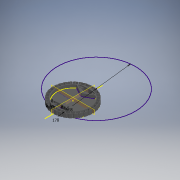
# Autodesk Inventor part: tsop_lid_edge
Saved by Autodesk Inventor 2020 (Build 240168000, 168)
## iProperties
Created: 2024-11-04
Part Number: tsop_lid_edge
Material: Полиэтилен, низкая плотность
Document SubType Name: Modeling
Designer: Ivan
Density: 0.894 g/cm^3
Appearance: Типовые
Mass: 25.9843 g
Surface Area: 265.893 cm^2
Volume: 29.0652 cm^3
Author: Ivan
Autodesk Inventor part; units mm, degrees
ref_plane "XZ Plane" through (0, 0, 0) normal (0, 1, 0) x (-1, 0, 0)
sketch "Эскиз1" plane through (0, 0, 0) normal (0, 1, 0) x (-1, 0, 0)
  line L0 (44.0469, 3.6) -> (38.8469, 3.6)
  line L1 (38.8469, 3.6) -> (38.8469, -3.6)
  line L2 (38.8469, -3.6) -> (44.0469, -3.6)
  line L3 (44.0469, -3.6) -> (44.0469, 3.6)
  line L4 (0, 0) -> (38.8469, 0) construction
  circle A0 centre (0, 0) radius 41.603 construction
  line L5 (41.4469, 3.6) -> (41.4469, -3.6) construction
  line L6 (37.3982, 11.1095) -> (38.8028, 4.0478)
  line L7 (42.4983, 12.124) -> (37.3982, 11.1095)
  line L8 (43.9029, 5.0623) -> (42.4983, 12.124)
  line L9 (38.8028, 4.0478) -> (43.9029, 5.0623)
  line L10 (34.5122, 18.192) -> (37.2675, 11.5401)
  line L11 (39.3164, 20.182) -> (34.5122, 18.192)
  line L12 (42.0717, 13.5301) -> (39.3164, 20.182)
  line L13 (37.2675, 11.5401) -> (42.0717, 13.5301)
  line L14 (30.3, 24.5755) -> (34.3001, 18.5889)
  line L15 (34.6236, 27.4645) -> (30.3, 24.5755)
  line L16 (38.6237, 21.4779) -> (34.6236, 27.4645)
  line L17 (34.3001, 18.5889) -> (38.6237, 21.4779)
  line L18 (24.9233, 30.0145) -> (30.0145, 24.9233)
  line L19 (28.6003, 33.6915) -> (24.9233, 30.0145)
  line L20 (33.6915, 28.6003) -> (28.6003, 33.6915)
  line L21 (30.0145, 24.9233) -> (33.6915, 28.6003)
  line L22 (18.5889, 34.3001) -> (24.5755, 30.3)
  line L23 (21.4779, 38.6237) -> (18.5889, 34.3001)
  line L24 (27.4645, 34.6236) -> (21.4779, 38.6237)
  line L25 (24.5755, 30.3) -> (27.4645, 34.6236)
  line L26 (11.5401, 37.2675) -> (18.192, 34.5122)
  line L27 (13.5301, 42.0717) -> (11.5401, 37.2675)
  line L28 (20.182, 39.3164) -> (13.5301, 42.0717)
  line L29 (18.192, 34.5122) -> (20.182, 39.3164)
  line L30 (4.0478, 38.8028) -> (11.1095, 37.3982)
  line L31 (5.0623, 43.9029) -> (4.0478, 38.8028)
  line L32 (12.124, 42.4983) -> (5.0623, 43.9029)
  line L33 (11.1095, 37.3982) -> (12.124, 42.4983)
  line L34 (-3.6, 38.8469) -> (3.6, 38.8469)
  line L35 (-3.6, 44.0469) -> (-3.6, 38.8469)
  line L36 (3.6, 44.0469) -> (-3.6, 44.0469)
  line L37 (3.6, 38.8469) -> (3.6, 44.0469)
  line L38 (-11.1095, 37.3982) -> (-4.0478, 38.8028)
  line L39 (-12.124, 42.4983) -> (-11.1095, 37.3982)
  line L40 (-5.0623, 43.9029) -> (-12.124, 42.4983)
  line L41 (-4.0478, 38.8028) -> (-5.0623, 43.9029)
  line L42 (-18.192, 34.5122) -> (-11.5401, 37.2675)
  line L43 (-20.182, 39.3164) -> (-18.192, 34.5122)
  line L44 (-13.5301, 42.0717) -> (-20.182, 39.3164)
  line L45 (-11.5401, 37.2675) -> (-13.5301, 42.0717)
  line L46 (-24.5755, 30.3) -> (-18.5889, 34.3001)
  line L47 (-27.4645, 34.6236) -> (-24.5755, 30.3)
  line L48 (-21.4779, 38.6237) -> (-27.4645, 34.6236)
  line L49 (-18.5889, 34.3001) -> (-21.4779, 38.6237)
  line L50 (-30.0145, 24.9233) -> (-24.9233, 30.0145)
  line L51 (-33.6915, 28.6003) -> (-30.0145, 24.9233)
  line L52 (-28.6003, 33.6915) -> (-33.6915, 28.6003)
  line L53 (-24.9233, 30.0145) -> (-28.6003, 33.6915)
  line L54 (-34.3001, 18.5889) -> (-30.3, 24.5755)
  line L55 (-38.6237, 21.4779) -> (-34.3001, 18.5889)
  line L56 (-34.6236, 27.4645) -> (-38.6237, 21.4779)
  line L57 (-30.3, 24.5755) -> (-34.6236, 27.4645)
  line L58 (-37.2675, 11.5401) -> (-34.5122, 18.192)
  line L59 (-42.0717, 13.5301) -> (-37.2675, 11.5401)
  line L60 (-39.3164, 20.182) -> (-42.0717, 13.5301)
  line L61 (-34.5122, 18.192) -> (-39.3164, 20.182)
  line L62 (-38.8028, 4.0478) -> (-37.3982, 11.1095)
  line L63 (-43.9029, 5.0623) -> (-38.8028, 4.0478)
  line L64 (-42.4983, 12.124) -> (-43.9029, 5.0623)
  line L65 (-37.3982, 11.1095) -> (-42.4983, 12.124)
  line L66 (-38.8469, -3.6) -> (-38.8469, 3.6)
  line L67 (-44.0469, -3.6) -> (-38.8469, -3.6)
  line L68 (-44.0469, 3.6) -> (-44.0469, -3.6)
  line L69 (-38.8469, 3.6) -> (-44.0469, 3.6)
  line L70 (-37.3982, -11.1095) -> (-38.8028, -4.0478)
  line L71 (-42.4983, -12.124) -> (-37.3982, -11.1095)
  line L72 (-43.9029, -5.0623) -> (-42.4983, -12.124)
  line L73 (-38.8028, -4.0478) -> (-43.9029, -5.0623)
  line L74 (-34.5122, -18.192) -> (-37.2675, -11.5401)
  line L75 (-39.3164, -20.182) -> (-34.5122, -18.192)
  line L76 (-42.0717, -13.5301) -> (-39.3164, -20.182)
  line L77 (-37.2675, -11.5401) -> (-42.0717, -13.5301)
  line L78 (-30.3, -24.5755) -> (-34.3001, -18.5889)
  line L79 (-34.6236, -27.4645) -> (-30.3, -24.5755)
  line L80 (-38.6237, -21.4779) -> (-34.6236, -27.4645)
  line L81 (-34.3001, -18.5889) -> (-38.6237, -21.4779)
  line L82 (-24.9233, -30.0145) -> (-30.0145, -24.9233)
  line L83 (-28.6003, -33.6915) -> (-24.9233, -30.0145)
  line L84 (-33.6915, -28.6003) -> (-28.6003, -33.6915)
  line L85 (-30.0145, -24.9233) -> (-33.6915, -28.6003)
  line L86 (-18.5889, -34.3001) -> (-24.5755, -30.3)
  line L87 (-21.4779, -38.6237) -> (-18.5889, -34.3001)
  line L88 (-27.4645, -34.6236) -> (-21.4779, -38.6237)
  line L89 (-24.5755, -30.3) -> (-27.4645, -34.6236)
  line L90 (-11.5401, -37.2675) -> (-18.192, -34.5122)
  line L91 (-13.5301, -42.0717) -> (-11.5401, -37.2675)
  line L92 (-20.182, -39.3164) -> (-13.5301, -42.0717)
  line L93 (-18.192, -34.5122) -> (-20.182, -39.3164)
  line L94 (-4.0478, -38.8028) -> (-11.1095, -37.3982)
  line L95 (-5.0623, -43.9029) -> (-4.0478, -38.8028)
  line L96 (-12.124, -42.4983) -> (-5.0623, -43.9029)
  line L97 (-11.1095, -37.3982) -> (-12.124, -42.4983)
  line L98 (3.6, -38.8469) -> (-3.6, -38.8469)
  line L99 (3.6, -44.0469) -> (3.6, -38.8469)
  line L100 (-3.6, -44.0469) -> (3.6, -44.0469)
  line L101 (-3.6, -38.8469) -> (-3.6, -44.0469)
  line L102 (11.1095, -37.3982) -> (4.0478, -38.8028)
  line L103 (12.124, -42.4983) -> (11.1095, -37.3982)
  line L104 (5.0623, -43.9029) -> (12.124, -42.4983)
  line L105 (4.0478, -38.8028) -> (5.0623, -43.9029)
  line L106 (18.192, -34.5122) -> (11.5401, -37.2675)
  line L107 (20.182, -39.3164) -> (18.192, -34.5122)
  line L108 (13.5301, -42.0717) -> (20.182, -39.3164)
  line L109 (11.5401, -37.2675) -> (13.5301, -42.0717)
  line L110 (24.5755, -30.3) -> (18.5889, -34.3001)
  line L111 (27.4645, -34.6236) -> (24.5755, -30.3)
  line L112 (21.4779, -38.6237) -> (27.4645, -34.6236)
  line L113 (18.5889, -34.3001) -> (21.4779, -38.6237)
  line L114 (30.0145, -24.9233) -> (24.9233, -30.0145)
  line L115 (33.6915, -28.6003) -> (30.0145, -24.9233)
  line L116 (28.6003, -33.6915) -> (33.6915, -28.6003)
  line L117 (24.9233, -30.0145) -> (28.6003, -33.6915)
  line L118 (34.3001, -18.5889) -> (30.3, -24.5755)
  line L119 (38.6237, -21.4779) -> (34.3001, -18.5889)
  line L120 (34.6236, -27.4645) -> (38.6237, -21.4779)
  line L121 (30.3, -24.5755) -> (34.6236, -27.4645)
  line L122 (37.2675, -11.5401) -> (34.5122, -18.192)
  line L123 (42.0717, -13.5301) -> (37.2675, -11.5401)
  line L124 (39.3164, -20.182) -> (42.0717, -13.5301)
  line L125 (34.5122, -18.192) -> (39.3164, -20.182)
  line L126 (38.8028, -4.0478) -> (37.3982, -11.1095)
  line L127 (43.9029, -5.0623) -> (38.8028, -4.0478)
  line L128 (42.4983, -12.124) -> (43.9029, -5.0623)
  line L129 (37.3982, -11.1095) -> (42.4983, -12.124)
  line L130 (38.8028, 4.0478) -> (38.8469, 3.6) construction
  line L131 (38.8469, 3.6) -> (43.9777, 4.1053) construction
  line L132 (43.9029, 5.0623) -> (37.3982, 11.1095) construction
  line L133 (42.4983, 12.124) -> (38.8028, 4.0478) construction
  circle A1 centre (0, 0) radius 41.4469 construction
  line L134 (39.3164, 20.182) -> (37.2675, 11.5401) construction
  line L135 (34.5122, 18.192) -> (42.0717, 13.5301) construction
  line L136 (38.292, 15.8611) -> (0, 0) construction
  line L137 (0, 0) -> (40.6505, 8.0859) construction
  point P0 (41.603, 0)
  point P1 (38.1005, 7.5787)
  point P2 (39.9482, 11.6167)
  point P3 (41.3529, 4.5551)
  point P4 (35.8899, 14.8661)
  point P5 (36.9143, 19.187)
  point P6 (39.6696, 12.5351)
  point P7 (32.3, 21.5822)
  point P8 (32.4618, 26.02)
  point P9 (36.4619, 20.0334)
  point P10 (27.4689, 27.4689)
  point P11 (26.7618, 31.853)
  point P12 (31.853, 26.7618)
  point P13 (21.5822, 32.3)
  point P14 (20.0334, 36.4619)
  point P15 (26.02, 32.4618)
  point P16 (14.8661, 35.8899)
  point P17 (12.5351, 39.6696)
  point P18 (19.187, 36.9143)
  point P19 (7.5787, 38.1005)
  point P20 (4.5551, 41.3529)
  point P21 (11.6167, 39.9482)
  point P22 (0, 38.8469)
  point P23 (-3.6, 41.4469)
  point P24 (3.6, 41.4469)
  point P25 (-7.5787, 38.1005)
  point P26 (-11.6167, 39.9482)
  point P27 (-4.5551, 41.3529)
  point P28 (-14.8661, 35.8899)
  point P29 (-19.187, 36.9143)
  point P30 (-12.5351, 39.6696)
  point P31 (-21.5822, 32.3)
  point P32 (-26.02, 32.4618)
  point P33 (-20.0334, 36.4619)
  point P34 (-27.4689, 27.4689)
  point P35 (-31.853, 26.7618)
  point P36 (-26.7618, 31.853)
  point P37 (-32.3, 21.5822)
  point P38 (-36.4619, 20.0334)
  point P39 (-32.4618, 26.02)
  point P40 (-35.8899, 14.8661)
  point P41 (-39.6696, 12.5351)
  point P42 (-36.9143, 19.187)
  point P43 (-38.1005, 7.5787)
  point P44 (-41.3529, 4.5551)
  point P45 (-39.9482, 11.6167)
  point P46 (-38.8469, 0)
  point P47 (-41.4469, -3.6)
  point P48 (-41.4469, 3.6)
  point P49 (-38.1005, -7.5787)
  point P50 (-39.9482, -11.6167)
  point P51 (-41.3529, -4.5551)
  point P52 (-35.8899, -14.8661)
  point P53 (-36.9143, -19.187)
  point P54 (-39.6696, -12.5351)
  point P55 (-32.3, -21.5822)
  point P56 (-32.4618, -26.02)
  point P57 (-36.4619, -20.0334)
  point P58 (-27.4689, -27.4689)
  point P59 (-26.7618, -31.853)
  point P60 (-31.853, -26.7618)
  point P61 (-21.5822, -32.3)
  point P62 (-20.0334, -36.4619)
  point P63 (-26.02, -32.4618)
  point P64 (-14.8661, -35.8899)
  point P65 (-12.5351, -39.6696)
  point P66 (-19.187, -36.9143)
  point P67 (-7.5787, -38.1005)
  point P68 (-4.5551, -41.3529)
  point P69 (-11.6167, -39.9482)
  point P70 (0, -38.8469)
  point P71 (3.6, -41.4469)
  point P72 (-3.6, -41.4469)
  point P73 (7.5787, -38.1005)
  point P74 (11.6167, -39.9482)
  point P75 (4.5551, -41.3529)
  point P76 (14.8661, -35.8899)
  point P77 (19.187, -36.9143)
  point P78 (12.5351, -39.6696)
  point P79 (21.5822, -32.3)
  point P80 (26.02, -32.4618)
  point P81 (20.0334, -36.4619)
  point P82 (27.4689, -27.4689)
  point P83 (31.853, -26.7618)
  point P84 (26.7618, -31.853)
  point P85 (32.3, -21.5822)
  point P86 (36.4619, -20.0334)
  point P87 (32.4618, -26.02)
  point P88 (35.8899, -14.8661)
  point P89 (39.6696, -12.5351)
  point P90 (36.9143, -19.187)
  point P91 (38.1005, -7.5787)
  point P92 (41.3529, -4.5551)
  point P93 (39.9482, -11.6167)
  dimension "d79" = 82.8939
  dimension "d0" = 7.2
  dimension "d1" = 5.2
  dimension "d5" = 360
  dimension "d7" = 0.45
  dimension "d80" = 7.2
  dimension "d81" = 5.2
  dimension "d82" = 11.25
  dimension "d83" = 11.25
  constraints: 274 end point, 35 midpoint, 3 point on circle, 2 coincident, 2 horizontal, 2 perpendicular, 1 centre point, 1 parallel, 1 point on line, 1 vertical, 360 other
  measures "d0" distance of L1.start L1.end
  measures "d1" distance from line of L1 L2.end
  measures "d7" distance from line of L131 L6.end
  measures "d80" distance between parallel lines of L9 L7
  measures "d81" distance between parallel lines of L6 L8
  measures "d82" angle to the sketch x axis of L9
  measures "d83" angle of L137 L136
sketch "Эскиз3" plane through (0, 0, 0) normal (0, 1, 0) x (-1, 0, 0)
  line L0 (38.8028, 4.0478) -> (38.8469, 3.6) construction
  line L1 (38.8249, 3.8239) -> (46.4311, 4.5731) construction
  line L2 (44.0469, -3.6) -> (44.0469, 3.6) projected
  line L3 (44.0469, -0.05) -> (44.0469, 0.05)
  line L4 (44.0469, 2.45) -> (45.2469, 2.45) construction
  arc A0 (44.0469, 0.05) -> (45.2469, 2.45) centre (42.2469, 2.45) ccw
  line L5 (45.2469, 2.45) -> (45.2469, 0) construction
  line L6 (0, 0) -> (38.8469, 0) construction
  arc A1 (45.2469, -2.45) -> (44.0469, -0.05) centre (42.2469, -2.45) ccw
  arc A2 (43.1908, 8.6422) -> (43.8996, 11.2302) centre (40.9572, 10.6449) ccw
  arc A3 (44.8555, 6.4243) -> (43.2103, 8.5441) centre (41.9131, 5.839) ccw
  line L7 (43.2103, 8.5441) -> (43.1908, 8.6422)
  arc A4 (40.6749, 16.9022) -> (40.8651, 19.5788) centre (38.0935, 18.4307) ccw
  arc A5 (42.7403, 15.0517) -> (40.7132, 16.8098) centre (39.9686, 13.9037) ccw
  line L8 (40.7132, 16.8098) -> (40.6749, 16.9022)
  arc A6 (36.5959, 24.5127) -> (36.2603, 27.1749) centre (33.7659, 25.5082) ccw
  arc A7 (38.9826, 23.1007) -> (36.6515, 24.4296) centre (36.4882, 21.434) ccw
  line L9 (36.6515, 24.4296) -> (36.5959, 24.5127)
  arc A8 (31.1105, 31.1812) -> (30.262, 33.7268) centre (28.1407, 31.6055) ccw
  arc A9 (33.7268, 30.262) -> (31.1812, 31.1105) centre (31.6055, 28.1407) ccw
  line L10 (31.1812, 31.1105) -> (31.1105, 31.1812)
  arc A10 (24.4296, 36.6515) -> (23.1007, 38.9826) centre (21.434, 36.4882) ccw
  arc A11 (27.1749, 36.2603) -> (24.5127, 36.5959) centre (25.5082, 33.7659) ccw
  line L11 (24.5127, 36.5959) -> (24.4296, 36.6515)
  arc A12 (16.8098, 40.7132) -> (15.0517, 42.7403) centre (13.9037, 39.9686) ccw
  arc A13 (19.5788, 40.8651) -> (16.9022, 40.6749) centre (18.4307, 38.0935) ccw
  line L12 (16.9022, 40.6749) -> (16.8098, 40.7132)
  arc A14 (8.5441, 43.2103) -> (6.4243, 44.8555) centre (5.839, 41.9131) ccw
  arc A15 (11.2302, 43.8996) -> (8.6422, 43.1908) centre (10.6449, 40.9572) ccw
  line L13 (8.6422, 43.1908) -> (8.5441, 43.2103)
  arc A16 (-0.05, 44.0469) -> (-2.45, 45.2469) centre (-2.45, 42.2469) ccw
  arc A17 (2.45, 45.2469) -> (0.05, 44.0469) centre (2.45, 42.2469) ccw
  line L14 (0.05, 44.0469) -> (-0.05, 44.0469)
  arc A18 (-8.6422, 43.1908) -> (-11.2302, 43.8996) centre (-10.6449, 40.9572) ccw
  arc A19 (-6.4243, 44.8555) -> (-8.5441, 43.2103) centre (-5.839, 41.9131) ccw
  line L15 (-8.5441, 43.2103) -> (-8.6422, 43.1908)
  arc A20 (-16.9022, 40.6749) -> (-19.5788, 40.8651) centre (-18.4307, 38.0935) ccw
  arc A21 (-15.0517, 42.7403) -> (-16.8098, 40.7132) centre (-13.9037, 39.9686) ccw
  line L16 (-16.8098, 40.7132) -> (-16.9022, 40.6749)
  arc A22 (-24.5127, 36.5959) -> (-27.1749, 36.2603) centre (-25.5082, 33.7659) ccw
  arc A23 (-23.1007, 38.9826) -> (-24.4296, 36.6515) centre (-21.434, 36.4882) ccw
  line L17 (-24.4296, 36.6515) -> (-24.5127, 36.5959)
  arc A24 (-31.1812, 31.1105) -> (-33.7268, 30.262) centre (-31.6055, 28.1407) ccw
  arc A25 (-30.262, 33.7268) -> (-31.1105, 31.1812) centre (-28.1407, 31.6055) ccw
  line L18 (-31.1105, 31.1812) -> (-31.1812, 31.1105)
  arc A26 (-36.6515, 24.4296) -> (-38.9826, 23.1007) centre (-36.4882, 21.434) ccw
  arc A27 (-36.2603, 27.1749) -> (-36.5959, 24.5127) centre (-33.7659, 25.5082) ccw
  line L19 (-36.5959, 24.5127) -> (-36.6515, 24.4296)
  arc A28 (-40.7132, 16.8098) -> (-42.7403, 15.0517) centre (-39.9686, 13.9037) ccw
  arc A29 (-40.8651, 19.5788) -> (-40.6749, 16.9022) centre (-38.0935, 18.4307) ccw
  line L20 (-40.6749, 16.9022) -> (-40.7132, 16.8098)
  arc A30 (-43.2103, 8.5441) -> (-44.8555, 6.4243) centre (-41.9131, 5.839) ccw
  arc A31 (-43.8996, 11.2302) -> (-43.1908, 8.6422) centre (-40.9572, 10.6449) ccw
  line L21 (-43.1908, 8.6422) -> (-43.2103, 8.5441)
  arc A32 (-44.0469, -0.05) -> (-45.2469, -2.45) centre (-42.2469, -2.45) ccw
  arc A33 (-45.2469, 2.45) -> (-44.0469, 0.05) centre (-42.2469, 2.45) ccw
  line L22 (-44.0469, 0.05) -> (-44.0469, -0.05)
  arc A34 (-43.1908, -8.6422) -> (-43.8996, -11.2302) centre (-40.9572, -10.6449) ccw
  arc A35 (-44.8555, -6.4243) -> (-43.2103, -8.5441) centre (-41.9131, -5.839) ccw
  line L23 (-43.2103, -8.5441) -> (-43.1908, -8.6422)
  arc A36 (-40.6749, -16.9022) -> (-40.8651, -19.5788) centre (-38.0935, -18.4307) ccw
  arc A37 (-42.7403, -15.0517) -> (-40.7132, -16.8098) centre (-39.9686, -13.9037) ccw
  line L24 (-40.7132, -16.8098) -> (-40.6749, -16.9022)
  arc A38 (-36.5959, -24.5127) -> (-36.2603, -27.1749) centre (-33.7659, -25.5082) ccw
  arc A39 (-38.9826, -23.1007) -> (-36.6515, -24.4296) centre (-36.4882, -21.434) ccw
  line L25 (-36.6515, -24.4296) -> (-36.5959, -24.5127)
  arc A40 (-31.1105, -31.1812) -> (-30.262, -33.7268) centre (-28.1407, -31.6055) ccw
  arc A41 (-33.7268, -30.262) -> (-31.1812, -31.1105) centre (-31.6055, -28.1407) ccw
  line L26 (-31.1812, -31.1105) -> (-31.1105, -31.1812)
  arc A42 (-24.4296, -36.6515) -> (-23.1007, -38.9826) centre (-21.434, -36.4882) ccw
  arc A43 (-27.1749, -36.2603) -> (-24.5127, -36.5959) centre (-25.5082, -33.7659) ccw
  line L27 (-24.5127, -36.5959) -> (-24.4296, -36.6515)
  arc A44 (-16.8098, -40.7132) -> (-15.0517, -42.7403) centre (-13.9037, -39.9686) ccw
  arc A45 (-19.5788, -40.8651) -> (-16.9022, -40.6749) centre (-18.4307, -38.0935) ccw
  line L28 (-16.9022, -40.6749) -> (-16.8098, -40.7132)
  arc A46 (-8.5441, -43.2103) -> (-6.4243, -44.8555) centre (-5.839, -41.9131) ccw
  arc A47 (-11.2302, -43.8996) -> (-8.6422, -43.1908) centre (-10.6449, -40.9572) ccw
  line L29 (-8.6422, -43.1908) -> (-8.5441, -43.2103)
  arc A48 (0.05, -44.0469) -> (2.45, -45.2469) centre (2.45, -42.2469) ccw
  arc A49 (-2.45, -45.2469) -> (-0.05, -44.0469) centre (-2.45, -42.2469) ccw
  line L30 (-0.05, -44.0469) -> (0.05, -44.0469)
  arc A50 (8.6422, -43.1908) -> (11.2302, -43.8996) centre (10.6449, -40.9572) ccw
  arc A51 (6.4243, -44.8555) -> (8.5441, -43.2103) centre (5.839, -41.9131) ccw
  line L31 (8.5441, -43.2103) -> (8.6422, -43.1908)
  arc A52 (16.9022, -40.6749) -> (19.5788, -40.8651) centre (18.4307, -38.0935) ccw
  arc A53 (15.0517, -42.7403) -> (16.8098, -40.7132) centre (13.9037, -39.9686) ccw
  line L32 (16.8098, -40.7132) -> (16.9022, -40.6749)
  arc A54 (24.5127, -36.5959) -> (27.1749, -36.2603) centre (25.5082, -33.7659) ccw
  arc A55 (23.1007, -38.9826) -> (24.4296, -36.6515) centre (21.434, -36.4882) ccw
  line L33 (24.4296, -36.6515) -> (24.5127, -36.5959)
  arc A56 (31.1812, -31.1105) -> (33.7268, -30.262) centre (31.6055, -28.1407) ccw
  arc A57 (30.262, -33.7268) -> (31.1105, -31.1812) centre (28.1407, -31.6055) ccw
  line L34 (31.1105, -31.1812) -> (31.1812, -31.1105)
  arc A58 (36.6515, -24.4296) -> (38.9826, -23.1007) centre (36.4882, -21.434) ccw
  arc A59 (36.2603, -27.1749) -> (36.5959, -24.5127) centre (33.7659, -25.5082) ccw
  line L35 (36.5959, -24.5127) -> (36.6515, -24.4296)
  arc A60 (40.7132, -16.8098) -> (42.7403, -15.0517) centre (39.9686, -13.9037) ccw
  arc A61 (40.8651, -19.5788) -> (40.6749, -16.9022) centre (38.0935, -18.4307) ccw
  line L36 (40.6749, -16.9022) -> (40.7132, -16.8098)
  arc A62 (43.2103, -8.5441) -> (44.8555, -6.4243) centre (41.9131, -5.839) ccw
  arc A63 (43.8996, -11.2302) -> (43.1908, -8.6422) centre (40.9572, -10.6449) ccw
  line L37 (43.1908, -8.6422) -> (43.2103, -8.5441)
  arc A64 (45.2469, 2.45) -> (44.8555, 6.4243) centre (0, 0) ccw
  arc A65 (43.8996, 11.2302) -> (42.7403, 15.0517) centre (0, 0) ccw
  arc A66 (40.8651, 19.5788) -> (38.9826, 23.1007) centre (0, 0) ccw
  arc A67 (36.2603, 27.1749) -> (33.7268, 30.262) centre (0, 0) ccw
  arc A68 (30.262, 33.7268) -> (27.1749, 36.2603) centre (0, 0) ccw
  arc A69 (23.1007, 38.9826) -> (19.5788, 40.8651) centre (0, 0) ccw
  arc A70 (15.0517, 42.7403) -> (11.2302, 43.8996) centre (0, 0) ccw
  arc A71 (6.4243, 44.8555) -> (2.45, 45.2469) centre (0, 0) ccw
  arc A72 (-2.45, 45.2469) -> (-6.4243, 44.8555) centre (0, 0) ccw
  arc A73 (-11.2302, 43.8996) -> (-15.0517, 42.7403) centre (0, 0) ccw
  arc A74 (-19.5788, 40.8651) -> (-23.1007, 38.9826) centre (0, 0) ccw
  arc A75 (-27.1749, 36.2603) -> (-30.262, 33.7268) centre (0, 0) ccw
  arc A76 (-33.7268, 30.262) -> (-36.2603, 27.1749) centre (0, 0) ccw
  arc A77 (-38.9826, 23.1007) -> (-40.8651, 19.5788) centre (0, 0) ccw
  arc A78 (-42.7403, 15.0517) -> (-43.8996, 11.2302) centre (0, 0) ccw
  arc A79 (-44.8555, 6.4243) -> (-45.2469, 2.45) centre (0, 0) ccw
  arc A80 (-45.2469, -2.45) -> (-44.8555, -6.4243) centre (0, 0) ccw
  arc A81 (-43.8996, -11.2302) -> (-42.7403, -15.0517) centre (0, 0) ccw
  arc A82 (-40.8651, -19.5788) -> (-38.9826, -23.1007) centre (0, 0) ccw
  arc A83 (-36.2603, -27.1749) -> (-33.7268, -30.262) centre (0, 0) ccw
  arc A84 (-30.262, -33.7268) -> (-27.1749, -36.2603) centre (0, 0) ccw
  arc A85 (-23.1007, -38.9826) -> (-19.5788, -40.8651) centre (0, 0) ccw
  arc A86 (-15.0517, -42.7403) -> (-11.2302, -43.8996) centre (0, 0) ccw
  arc A87 (-6.4243, -44.8555) -> (-2.45, -45.2469) centre (0, 0) ccw
  arc A88 (2.45, -45.2469) -> (6.4243, -44.8555) centre (0, 0) ccw
  arc A89 (11.2302, -43.8996) -> (15.0517, -42.7403) centre (0, 0) ccw
  arc A90 (19.5788, -40.8651) -> (23.1007, -38.9826) centre (0, 0) ccw
  arc A91 (27.1749, -36.2603) -> (30.262, -33.7268) centre (0, 0) ccw
  arc A92 (33.7268, -30.262) -> (36.2603, -27.1749) centre (0, 0) ccw
  arc A93 (38.9826, -23.1007) -> (40.8651, -19.5788) centre (0, 0) ccw
  arc A94 (42.7403, -15.0517) -> (43.8996, -11.2302) centre (0, 0) ccw
  arc A95 (44.8555, -6.4243) -> (45.2469, -2.45) centre (0, 0) ccw
  circle A96 centre (0, 0) radius 36.8469
  line L38 (38.8469, 3.6) -> (38.8469, -3.6) projected
  point P0 (44.0469, 0)
  point P1 (43.2006, 8.5931)
  point P2 (40.6941, 16.856)
  point P3 (36.6237, 24.4712)
  point P4 (31.1459, 31.1459)
  point P5 (24.4712, 36.6237)
  point P6 (16.856, 40.6941)
  point P7 (8.5931, 43.2006)
  point P8 (0, 44.0469)
  point P9 (-8.5931, 43.2006)
  point P10 (-16.856, 40.6941)
  point P11 (-24.4712, 36.6237)
  point P12 (-31.1459, 31.1459)
  point P13 (-36.6237, 24.4712)
  point P14 (-40.6941, 16.856)
  point P15 (-43.2006, 8.5931)
  point P16 (-44.0469, 0)
  point P17 (-43.2006, -8.5931)
  point P18 (-40.6941, -16.856)
  point P19 (-36.6237, -24.4712)
  point P20 (-31.1459, -31.1459)
  point P21 (-24.4712, -36.6237)
  point P22 (-16.856, -40.6941)
  point P23 (-8.5931, -43.2006)
  point P24 (0, -44.0469)
  point P25 (8.5931, -43.2006)
  point P26 (16.856, -40.6941)
  point P27 (24.4712, -36.6237)
  point P28 (31.1459, -31.1459)
  point P29 (36.6237, -24.4712)
  point P30 (40.6941, -16.856)
  point P31 (43.2006, -8.5931)
  point P32 (36.8469, 0)
  point P33 (44.8555, -6.4243)
  point P34 (45.2469, -2.45)
  point P35 (44.0469, -0.05)
  point P36 (44.0469, 0.05)
  point P37 (43.8996, 11.2302)
  point P38 (42.7403, 15.0517)
  point P39 (40.8651, 19.5788)
  point P40 (38.9826, 23.1007)
  point P41 (36.2603, 27.1749)
  point P42 (33.7268, 30.262)
  point P43 (30.262, 33.7268)
  point P44 (27.1749, 36.2603)
  point P45 (23.1007, 38.9826)
  point P46 (19.5788, 40.8651)
  point P47 (15.0517, 42.7403)
  point P48 (11.2302, 43.8996)
  point P49 (6.4243, 44.8555)
  point P50 (2.45, 45.2469)
  point P51 (-2.45, 45.2469)
  point P52 (-6.4243, 44.8555)
  point P53 (-11.2302, 43.8996)
  point P54 (-15.0517, 42.7403)
  point P55 (-19.5788, 40.8651)
  point P56 (-23.1007, 38.9826)
  point P57 (-27.1749, 36.2603)
  point P58 (-30.262, 33.7268)
  point P59 (-33.7268, 30.262)
  point P60 (-36.2603, 27.1749)
  point P61 (-38.9826, 23.1007)
  point P62 (-40.8651, 19.5788)
  point P63 (-42.7403, 15.0517)
  point P64 (-43.8996, 11.2302)
  point P65 (-44.8555, 6.4243)
  point P66 (-45.2469, 2.45)
  point P67 (-45.2469, -2.45)
  point P68 (-44.8555, -6.4243)
  point P69 (-43.8996, -11.2302)
  point P70 (-42.7403, -15.0517)
  point P71 (-40.8651, -19.5788)
  point P72 (-38.9826, -23.1007)
  point P73 (-36.2603, -27.1749)
  point P74 (-33.7268, -30.262)
  point P75 (-30.262, -33.7268)
  point P76 (-27.1749, -36.2603)
  point P77 (-23.1007, -38.9826)
  point P78 (-19.5788, -40.8651)
  point P79 (-15.0517, -42.7403)
  point P80 (-11.2302, -43.8996)
  point P81 (-6.4243, -44.8555)
  point P82 (-2.45, -45.2469)
  point P83 (2.45, -45.2469)
  point P84 (6.4243, -44.8555)
  point P85 (11.2302, -43.8996)
  point P86 (15.0517, -42.7403)
  point P87 (19.5788, -40.8651)
  point P88 (23.1007, -38.9826)
  point P89 (27.1749, -36.2603)
  point P90 (30.262, -33.7268)
  point P91 (33.7268, -30.262)
  point P92 (36.2603, -27.1749)
  point P93 (38.9826, -23.1007)
  point P94 (40.8651, -19.5788)
  point P95 (42.7403, -15.0517)
  point P96 (43.8996, -11.2302)
  dimension "d25" = 0.1
  dimension "d26" = 1.2
  dimension "d29" = 2.4
  dimension "d32" = 360
  dimension "d36" = 360
  dimension "d38" = 2
  constraints: 192 point on circle, 96 centre point, 70 end point, 4 point on line, 2 coincident, 2 midpoint, 2 perpendicular, 2 symmetric about line, 1 collinear, 1 horizontal, 1 horizontal alignment, 1 tangent, 453 other
  measures "d25" distance of L3.start L3.end
  measures "d26" distance of L4.start L4.end
  measures "d29" distance from line of L4 L3.end
  measures "d38" distance from line of L38 point (36.847, 0)
extrude "Выдавливание4" add sketch "Эскиз3" along normal blind 7.2
extrude "Выдавливание3" cut sketch "Эскиз1" along normal through all
extrude "Выдавливание5" add sketch "Эскиз3" against normal blind 2
sketch "Эскиз5" plane through (0, -2, 0) normal (0, -1, 0) x (1, 0, 0)
  circle A0 centre (0, 0) radius 36.8469 projected
  line L0 (-15.1, 31) -> (15.1, 31) construction
  line L1 (15.1, 31) -> (15.1, -31) construction
  line L2 (15.1, -31) -> (-15.1, -31) construction
  line L3 (-15.1, -31) -> (-15.1, 31) construction
  line L4 (15.1, -31) -> (-15.1, 31) construction
  circle A1 centre (-15.1, 31) radius 1.65
  circle A2 centre (15.1, 31) radius 1.65
  circle A3 centre (15.1, -31) radius 1.65
  circle A4 centre (-15.1, -31) radius 1.65
  line L5 (0, -31) -> (0, 31) construction
  circle A5 centre (0, -22.6275) radius 2
  circle A6 centre (0, 22.6275) radius 2
  dimension "d51" = 30.2
  dimension "d52" = 62
  dimension "d53" = 3.3
  dimension "d54" = 4
  dimension "d55" = 45.255
  dimension "d56" = 22.6275
  constraints: 12 end point, 6 centre point, 5 coincident, 4 equal radius, 4 midpoint, 2 parallel, 2 perpendicular, 2 point on line, 1 horizontal
  measures "d51" distance of L1.end L2.end
  measures "d52" distance of L0.end L1.end
  measures "d53" diameter of A1
  measures "d54" diameter of A5
  measures "d55" distance of A6.centre A5.centre
  measures "d56" distance of point (0, 0) A6.centre
extrude "Выдавливание6" add sketch "Эскиз5" against normal blind 2.5
chamfer "Фаска2" distance 1.4 angle 45 4 edges at (-16.75, -2, 31) (13.45, -2, -31) (-16.75, -2, -31) (13.45, -2, 31)
sketch "Эскиз7" plane through (0, 0.5, 0) normal (0, 1, 0) x (1, 0, 0)
  circle A0 centre (0, 0) radius 36.8469 projected
  circle A1 centre (15.1, -31) radius 1.65 projected
  circle A2 centre (0, -22.6275) radius 2 projected
  circle A3 centre (-15.1, -31) radius 1.65 projected
  circle A4 centre (-15.1, 31) radius 1.65 projected
  circle A5 centre (0, 22.6275) radius 2 projected
  circle A6 centre (15.1, 31) radius 1.65 projected
  circle A7 centre (-15.1, -31) radius 4 construction
  circle A8 centre (15.1, -31) radius 1.65 projected
  circle A9 centre (15.1, -31) radius 4 construction
  circle A10 centre (15.1, 31) radius 3.05 construction
  circle A11 centre (15.1, 31) radius 4 construction
  circle A12 centre (-15.1, 31) radius 1.65 projected
  circle A13 centre (-15.1, 31) radius 4 construction
  circle A14 centre (0, 0) radius 36.8469 projected
  line L0 (-13.073, -34.4498) -> (0, -27.2012)
  line L1 (-21.46, -29.9527) -> (-1.9397, -19.1293)
  line L2 (13.073, -34.4498) -> (-1.9397, -26.1257)
  line L3 (21.46, -29.9527) -> (1.9397, -19.1293)
  line L4 (-15.1, -31) -> (-9.8654, -28.0975) construction
  line L5 (15.1, -31) -> (8.9364, -27.5825) construction
  circle A15 centre (0, -22.6275) radius 4
  line L6 (0, 0) -> (-36.8469, 0) construction
  line L7 (-13.073, 34.4498) -> (0, 27.2012)
  line L8 (-21.46, 29.9527) -> (-1.9397, 19.1293)
  line L9 (13.073, 34.4498) -> (-1.9397, 26.1257)
  line L10 (21.46, 29.9527) -> (1.9397, 19.1293)
  circle A16 centre (0, 22.6275) radius 4
  circle A17 centre (-15.1, -31) radius 1.65 projected
  circle A18 centre (-15.1, -31) radius 3.05
  circle A19 centre (15.1, -31) radius 3.05
  circle A20 centre (15.1, 31) radius 3.05
  circle A21 centre (-15.1, 31) radius 3.05
  circle A22 centre (-15.1, -31) radius 3.05 projected
  point P0 (21.46, 29.9527)
  point P1 (-13.073, 34.4498)
  point P2 (-21.46, 29.9527)
  point P3 (-21.46, -29.9527)
  point P4 (-13.073, -34.4498)
  point P5 (13.073, -34.4498)
  point P6 (21.46, -29.9527)
  dimension "d63" = 8
  dimension "d64" = 8
  dimension "d68" = 6.1
  constraints: 22 end point, 11 point on circle, 10 centre point, 9 coincident, 9 symmetric about line, 6 equal radius, 4 parallel, 4 point on line, 4 tangent, 1 horizontal, 1 other
  measures "d63" diameter of A7
  measures "d64" diameter of A15
  measures "d68" diameter of A18
extrude "Выдавливание7" add sketch "Эскиз7" along normal up to surface (6.7 mm away) contours L10 A16 L9 A0 A20 | A0 A19 L2 A15 L3 | A16 | A15 | L8 A0 A21 L7 L9 A16 | A15 L2 L0 A0 A18 L1
fillet "Сопряжение1" radius 2 14 edges at (-13.073, 3.85, 34.4498) (13.073, 3.85, 34.4498) (0, 3.85, 27.2012) (1.9397, 3.85, 19.1293) (-1.9397, 3.85, 19.1293) (1.9397, 3.85, -19.1293) (0, 3.85, -27.2012) (-1.9397, 3.85, -19.1293) (-13.073, 3.85, -34.4498) (13.073, 3.85, -34.4498) (21.46, 3.85, -29.9527) (21.46, 3.85, 29.9527) (-21.46, 3.85, 29.9527) (-21.46, 3.85, -29.9527)
sketch "Эскиз10" plane through (0, 0.5, 0) normal (0, 1, 0) x (1, 0, 0)
  arc A0 (0.9698, -27.739) -> (-0.9698, -27.739) centre (0, -29.4881) ccw projected
  line L0 (-0.9698, -27.739) -> (-8.9601, -32.1694) projected
  arc A1 (-8.9601, -32.1694) -> (-8.4489, -35.8652) centre (-7.9903, -33.9185) ccw projected
  arc A2 (-8.4489, -35.8652) -> (8.4489, -35.8652) centre (0, 0) ccw projected
  arc A3 (8.4489, -35.8652) -> (8.9601, -32.1694) centre (7.9903, -33.9185) ccw projected
  line L1 (8.9601, -32.1694) -> (0.9698, -27.739) projected
  arc A4 (8.9601, 32.1694) -> (8.4489, 35.8652) centre (7.9903, 33.9185) ccw projected
  arc A5 (8.4489, 35.8652) -> (-8.4489, 35.8652) centre (0, 0) ccw projected
  arc A6 (-8.4489, 35.8652) -> (-8.9601, 32.1694) centre (-7.9903, 33.9185) ccw projected
  line L2 (-8.9601, 32.1694) -> (-0.9698, 27.739) projected
  arc A7 (-0.9698, 27.739) -> (0.9698, 27.739) centre (0, 29.4881) ccw projected
  line L3 (0.9698, 27.739) -> (8.9601, 32.1694) projected
extrude "Выдавливание8" cut sketch "Эскиз10" against normal up to surface (2.5 mm away)
sketch "Эскиз11" plane through (0, 7.2, 0) normal (0, 1, 0) x (1, 0, 0)
  circle A0 centre (0, -22.6275) radius 2 projected
  circle A1 centre (0, 22.6275) radius 2 projected
  point P0 (0, 0)
extrude "Выдавливание9" add sketch "Эскиз11" against normal blind 4.2
extrude "Выдавливание10" add sketch "Эскиз7" along normal blind 4.5 contours A20 A0 | A0 A20 | A19 A0 | A0 A19 | A21 A0 | A0 A21 | A18 A0 | A0 A18
sketch "Эскиз12" plane through (0, 7.2, 0) normal (0, 1, 0) x (1, 0, 0)
  arc A0 (-17.9014, 32.2062) -> (-14.3227, 33.9493) centre (-15.1, 31) ccw projected
  arc A1 (14.3227, 33.9493) -> (17.9014, 32.2062) centre (15.1, 31) ccw projected
  arc A2 (-14.3227, -33.9493) -> (-17.9014, -32.2062) centre (-15.1, -31) ccw projected
  arc A3 (17.9014, -32.2062) -> (14.3227, -33.9493) centre (15.1, -31) ccw projected
  arc A4 (-14.3227, 33.9493) -> (-17.9014, 32.2062) centre (-15.1, 31) ccw
  arc A5 (17.9014, 32.2062) -> (14.3227, 33.9493) centre (15.1, 31) ccw
  circle A6 centre (-15.1, -31) radius 1.65 projected
  arc A7 (-14.3227, -33.9493) -> (-17.9014, -32.2062) centre (-15.1, -31) ccw projected
  arc A8 (-17.9014, -32.2062) -> (-14.3227, -33.9493) centre (-15.1, -31) ccw
  arc A9 (14.3227, -33.9493) -> (17.9014, -32.2062) centre (15.1, -31) ccw
  line L0 (14.3227, -33.9493) -> (17.9014, -32.2062)
  line L1 (-14.3227, -33.9493) -> (-17.9014, -32.2062)
  line L2 (-17.9014, 32.2062) -> (-14.3227, 33.9493)
  arc A10 (17.9014, 32.2062) -> (14.3227, 33.9493) centre (0, 0) ccw projected
  line L3 (14.3227, 33.9493) -> (17.9014, 32.2062)
  constraints: 9 point on circle, 8 end point, 4 centre point, 4 coincident, 1 parallel
extrude "Выдавливание11" cut sketch "Эскиз12" against normal up to surface (2.2 mm away) contours A4 L2 | A5 A10 | A8 L1 | A9 L0
sketch "Эскиз15" plane through (0, -2, 0) normal (0, -1, 0) x (1, 0, 0)
  arc A0 (14.1508, 34.2546) -> (-13.0765, 34.4209) centre (0, -53.6132) ccw
  circle A1 centre (-15.1, 31) radius 3.05 projected
  circle A2 centre (15.1, 31) radius 3.05 projected
  arc A3 (-1.9397, 19.1293) -> (1.9397, 19.1293) centre (0, 22.6275) ccw projected
  circle A4 centre (0, -53.6132) radius 89
  line L0 (0, 25.8775) -> (-15.5093, 27.9776)
  line L1 (0, 25.8775) -> (15.5093, 27.9776)
  line L2 (0, 25.8775) -> (-13.5858, 33.6476) construction
  line L3 (0, 25.8775) -> (-12.832, 34.4569)
  arc A5 (-7.6106, 35.0608) -> (-7.7546, 26.9275) centre (-7.2609, 30.9867) ccw
  line L4 (0, 64.0889) -> (0, -67.8051) projected
  arc A6 (7.7546, 26.9275) -> (7.6106, 35.0608) centre (7.2609, 30.9867) ccw
  circle A7 centre (0, 22.6275) radius 3.25
  point P0 (0, 0)
  point P1 (0, 18.6275)
  point P2 (0.5435, 35.3851)
  point P3 (-7.8645, 26.9424)
  point P4 (7.7546, 26.9275)
  point P5 (7.6106, 35.0608)
  point P6 (-7.6106, 35.0608)
  dimension "d96" = 6.5
  dimension "d91" = 4
  dimension "d97" = 178
  dimension "d100" = 0.7
  constraints: 13 point on circle, 8 end point, 4 centre point, 4 tangent, 3 horizontal alignment, 2 coincident, 1 equal radius, 1 midpoint, 1 vertical alignment, 8 other
  measures "d91" angle of L3 L2
  measures "d97" diameter of A4
extrude "Выдавливание13" cut sketch "Эскиз15" against normal up to surface (9.2 mm away) contours A6 L1 L4 A0 | L4 L3 A5 A0 | L0 A5 L3
sketch "Эскиз16" plane through (0, 7.2, 0) normal (0, 1, 0) x (1, 0, 0)
  circle A0 centre (15.1, -31) radius 3.05 projected
  circle A1 centre (-15.1, -31) radius 3.05 projected
  line L0 (15.1, -31) -> (0, 0) construction
  circle A2 centre (-15.1, -31) radius 1.65 projected
  line L1 (0, 0) -> (-15.1, -31) construction
  line L2 (-15.1, -31) -> (-16.4356, -33.742) construction
  circle A3 centre (-15.1, -31) radius 3.05 projected
  line L3 (15.1, -31) -> (16.4356, -33.742) construction
  arc A4 (-22.5242, 29.1608) -> (-22.5242, -29.1608) centre (0, 0) ccw projected
  line L4 (15.1, -31) -> (8.9364, -27.5825) construction
  line L5 (15.1, -31) -> (15.5798, -27.988) construction
  circle A5 centre (15.1, -31) radius 3.05 projected
  line L6 (0, 63.3457) -> (0, -63.3457) projected
  line L7 (-15.1, -31) -> (-15.5798, -27.988) construction
  line L8 (0, -25.8775) -> (-7.8645, -26.9424) projected
  arc A6 (-16.4356, -33.742) -> (16.4356, -33.742) centre (0, 47.552) ccw
  line L9 (7.7546, -26.9275) -> (0, -25.8775) projected
  line L10 (7.7546, -26.9275) -> (15.5798, -27.988)
  line L11 (-7.8645, -26.9424) -> (-15.5798, -27.988)
  arc A7 (-13.0765, -34.4209) -> (14.1508, -34.2546) centre (0, 53.6132) ccw projected
  point P0 (0, -36.8469)
  point P1 (0, -26.6275)
  point P2 (0.0838, -35.3868)
  point P3 (-16.4356, -33.742)
  point P4 (14.8762, -34.0418)
  point P5 (15.4391, -27.9689)
  point P6 (-15.4391, -27.9689)
  point P7 (-14.8762, -34.0418)
  point P8 (0, -35.3868)
  dimension "d89" = 35.022
  dimension "d90" = 35.022
  constraints: 16 end point, 7 point on circle, 2 collinear, 2 symmetric about line, 1 centre point, 6 other
  measures "d89" angle of L4 L0
  measures "d90" angle of L0 L5
extrude "Выдавливание14" cut sketch "Эскиз16" against normal up to surface (2.2 mm away) contours A0 A6 L6 L9 L10 | A6 A1 L11 L8 L6
mirror "Зеркальное отражение1" about plane through (0, 0, 0) normal (0, 0, 1) of "Выдавливание13", "Выдавливание14"
sketch "Эскиз18" plane through (0, -2, 0) normal (0, -1, 0) x (1, 0, 0)
  arc A0 (8.4489, 35.8652) -> (-8.4489, 35.8652) centre (0, 0) ccw projected
  arc A1 (9.9869, 34.0346) -> (8.4489, 35.8652) centre (7.9903, 33.9185) ccw projected
  arc A2 (-8.4489, 35.8652) -> (-9.9869, 34.0346) centre (-7.9903, 33.9185) ccw projected
  arc A3 (7.7546, 26.9275) -> (7.6106, 35.0608) centre (7.2609, 30.9867) ccw projected
  arc A4 (14.1508, 34.2546) -> (-13.0765, 34.4209) centre (0, -53.6132) ccw projected
  arc A5 (-7.6106, 35.0608) -> (-7.7546, 26.9275) centre (-7.2609, 30.9867) ccw projected
  point P0 (9.7601, 34.85)
  point P1 (-9.7601, 34.85)
  point P2 (-9.7601, 34.85)
  point P3 (9.7601, 34.85)
extrude "Выдавливание15" add sketch "Эскиз18" against normal up to surface (9.2 mm away) contours A1 A4 A2 A0
extrude "Выдавливание16" add sketch "Эскиз18" against normal up to surface (7 mm away) contours A1 A3 A4 | A4 A5 A2
mirror "Зеркальное отражение2" about plane through (0, 0, 0) normal (0, 0, 1) of "Выдавливание15", "Выдавливание16"
fillet "Сопряжение2" radius 11 8 edges at (-14.8762, 6.1, -34.0418) (14.8762, 6.1, -34.0418) (0, 1.5, -25.8775) (0, 6.1, -25.8775) (-14.8762, 6.1, 34.0418) (14.8762, 6.1, 34.0418) (0, 1.5, 25.8775) (0, 6.1, 25.8775)
sketch "Эскиз19" plane through (0, -2, 0) normal (0, -1, 0) x (1, 0, 0)
  line L0 (-12.7849, -19.15) -> (-40, -19.15) projected
  line L1 (-9.4775, -19.15) -> (-3, -25.6275) projected
  line L2 (-3, -25.6275) -> (3, -25.6275) projected
  line L3 (3, -25.6275) -> (9.4775, -19.15) projected
  line L4 (-12.7849, 19.15) -> (-40, 19.15) projected
  line L5 (-3, 25.6275) -> (-9.4775, 19.15) projected
  line L6 (9.4775, 19.15) -> (3, 25.6275) projected
  line L7 (3, 25.6275) -> (-3, 25.6275) projected
  line L8 (40, 19.15) -> (2.5529, 19.15) projected
  line L9 (40, -19.15) -> (2.5529, -19.15) projected
  line L10 (40, -19.15) -> (40, 19.15) projected
  line L11 (-40, -19.15) -> (-40, 19.15) projected
  point P0 (0, 0)
equation "\"d29\" = 2 * d26"
equation "\"d56\" = 0.5 * d55"
equation "\"d64\" = d63"
